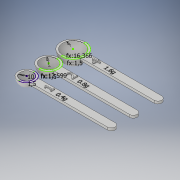
# Autodesk Inventor part: Pigmentlöffel
Saved by Autodesk Inventor 2018.2 (Build 222227000, 227)
## iProperties
Created: 2018-01-23
Part Number: Pigmentlöffel
Material: Generisch
Document SubType Name: Modeling
Designer: JochenAlt
Density: 1 g/cm^3
Appearance: Vorgabe
Author: JochenAlt
Autodesk Inventor part; units mm, degrees
ref_plane "XZ Plane" through (0, 0, 0) normal (0, 1, 0) x (-1, 0, 0)
ref_plane "XY Plane" through (0, 0, 0) normal (0, 0, 1) x (1, 0, 0)
sketch "Skizze1" plane through (0, 0, 0) normal (0, 0, 1) x (1, 0, 0)
  arc A0 (0, -5) -> (0, 5) centre (0, 0) ccw
  arc A1 (0, -6.5) -> (0, 6.5) centre (0, 0) ccw
  line L0 (0, -6.5) -> (0, -5)
  line L1 (0, 5) -> (0, 6.5)
  arc A2 (0, 11.07) -> (0, 23.669) centre (0, 17.3695) ccw
  arc A3 (0, 9.57) -> (0, 25.169) centre (0, 17.3695) ccw
  arc A4 (0, 28.5978) -> (0, 44.9639) centre (0, 36.7809) ccw
  arc A5 (0, 27.0978) -> (0, 46.4639) centre (0, 36.7809) ccw
  line L2 (0, 44.9639) -> (0, 46.4639)
  line L3 (0, 27.0978) -> (0, 28.5978)
  line L4 (0, 9.57) -> (0, 11.07)
  line L5 (0, 23.669) -> (0, 25.169)
  dimension "d0" = 10
  dimension "d8" = 1.5
  dimension "d9" = 12.599
  dimension "d10" = 1.5
  dimension "d11" = 16.3661
  dimension "d12" = 1.5
  constraints: 12 end point, 12 point on circle, 6 centre point, 6 vertical, 4 coincident
  measures "d0" diameter of A0
  measures "d8" radial gap between concentric circles of A1 A0
  measures "d9" diameter of A2
  measures "d10" radial gap between concentric circles of A3 A2
  measures "d11" diameter of A4
  measures "d12" radial gap between concentric circles of A5 A4
revolve "Umdrehung1" add sketch "Skizze1" angle 180 about axis through (0, -6.5, 0) along (0, 1, 0) contours A0 L1 A1 L0
revolve "Umdrehung2" add sketch "Skizze1" angle 180 about axis through (0, 9.57, 0) along (0, 1, 0) contours A2 L5 A3 L4
revolve "Umdrehung3" add sketch "Skizze1" angle 180 about axis through (0, 27.0978, 0) along (0, 1, 0) contours A4 L2 A5 L3
ref_plane "Arbeitsebene1" through (70, 0, 0) normal (1, 0, 0) x (0, 1, 0)
sketch "Skizze3" plane through (70, 0, 0) normal (1, 0, 0) x (0, 1, 0)
  line L0 (-5, 0) -> (5, 0) projected
  line L1 (-3, 0) -> (3, 0)
  line L2 (3, 0) -> (3, -2)
  line L3 (3, -2) -> (-3, -2)
  line L4 (-3, -2) -> (-3, 0)
  line L5 (14.3695, 0) -> (20.3695, 0)
  line L6 (20.3695, 0) -> (20.3695, -2)
  line L7 (20.3695, -2) -> (14.3695, -2)
  line L8 (14.3695, -2) -> (14.3695, 0)
  line L9 (33.7809, 0) -> (39.7809, 0)
  line L10 (39.7809, 0) -> (39.7809, -2)
  line L11 (39.7809, -2) -> (33.7809, -2)
  line L12 (33.7809, -2) -> (33.7809, 0)
  line L13 (25.169, 0) -> (9.57, 0) construction
  line L14 (46.4639, 0) -> (27.0978, 0) construction
  arc A0 (-5, 0) -> (5, 0) centre (0, 0) ccw construction
  line L15 (6.5, 0) -> (-6.5, 0) construction
  line L16 (0, 1.9354) -> (0, -11.6125) construction
  line L17 (-17.0928, 0) -> (57.0567, 0) construction
  line L18 (36.7809, 0) -> (36.7809, -9.6771) construction
  line L19 (17.3695, 0) -> (17.3695, -7.848) construction
  dimension "d16" = 2
  dimension "d17" = 6
  dimension "d21" = 6
  dimension "d22" = 6
  constraints: 28 end point, 6 parallel, 3 coincident, 3 horizontal, 3 perpendicular, 3 point on line, 2 collinear, 2 vertical, 4 other
  measures "d16" distance of the line from the sketch origin of L3
  measures "d17" distance between parallel lines of L2 L4
  measures "d21" distance between parallel lines of L6 L8
  measures "d22" distance between parallel lines of L10 L12
extrude "Extrusion2" add sketch "Skizze3" against normal up to next
fillet "Rundung1" radius 3 6 edges at (70, 3, -1) (70, -3, -1) (70, 14.3695, -1) (70, 20.3695, -1) (70, 33.7809, -1) (70, 39.7809, -1)
sketch "Skizze5" plane through (0, 0, 0) normal (0, 0, 1) x (1, 0, 0)
  line L0 (20.5874, 1.818) -> (20.5874, -1.1578)
  line L1 (20.5874, -1.1578) -> (19.9646, -1.1578)
  line L2 (19.9646, -1.1578) -> (19.9646, -0.0505)
  line L3 (19.9646, -0.0505) -> (15.8765, -0.0505)
  line L4 (15.8765, -0.0505) -> (15.8765, -1.1578)
  line L5 (15.8765, -1.1578) -> (15.3179, -1.1578)
  spline S0 degree 2 poles (15.3179, -1.1578) (15.3179, -0.53) (14.962, 0.0632) (14.4677, 0.1027) knots 0 0 0 1 2 2 2
  line L6 (14.4677, 0.1027) -> (14.4677, 0.7354)
  line L7 (14.4677, 0.7354) -> (19.9646, 0.7354)
  line L8 (19.9646, 0.7354) -> (19.9646, 1.818)
  line L9 (19.9646, 1.818) -> (20.5874, 1.818)
  line L10 (20.8624, 19.5576) -> (20.8624, 15.7958)
  line L11 (20.8624, 15.7958) -> (19.9973, 15.7958)
  spline S1 degree 2 poles (19.9973, 15.7958) (19.6167, 16.2012) (18.9098, 16.9229) (18.5292, 17.2689) knots 0 0 0 1 2 2 2
  spline S2 degree 2 poles (18.5292, 17.2689) (17.763, 17.9659) (16.8435, 18.4751) (16.3541, 18.4751) knots 0 0 0 1 2 2 2
  spline S3 degree 2 poles (16.3541, 18.4751) (16.0971, 18.4751) (15.7115, 18.3169) (15.5879, 18.1735) knots 0 0 0 1 2 2 2
  spline S4 degree 2 poles (15.5879, 18.1735) (15.4643, 18.0302) (15.3408, 17.6545) (15.3408, 17.4271) knots 0 0 0 1 2 2 2
  spline S5 degree 2 poles (15.3408, 17.4271) (15.3408, 17.2096) (15.4495, 16.7647) (15.5335, 16.562) knots 0 0 0 1 2 2 2
  spline S6 degree 2 poles (15.5335, 16.562) (15.6027, 16.389) (15.8005, 16.0677) (15.8697, 15.9688) knots 0 0 0 1 2 2 2
  line L12 (15.8697, 15.9688) -> (15.8697, 15.9243)
  line L13 (15.8697, 15.9243) -> (14.9997, 15.9243)
  spline S7 degree 2 poles (14.9997, 15.9243) (14.8761, 16.1764) (14.6339, 17.0811) (14.6339, 17.4864) knots 0 0 0 1 2 2 2
  spline S8 degree 2 poles (14.6339, 17.4864) (14.6339, 18.3416) (15.5385, 19.3055) (16.3096, 19.3055) knots 0 0 0 1 2 2 2
  spline S9 degree 2 poles (16.3096, 19.3055) (16.6705, 19.3055) (17.2736, 19.1375) (17.5306, 18.9892) knots 0 0 0 1 2 2 2
  spline S10 degree 2 poles (17.5306, 18.9892) (17.7976, 18.8409) (18.3215, 18.4108) (18.5737, 18.1735) knots 0 0 0 1 2 2 2
  spline S11 degree 2 poles (18.5737, 18.1735) (18.9938, 17.7879) (19.8935, 16.8438) (20.1555, 16.562) knots 0 0 0 1 2 2 2
  line L14 (20.1555, 16.562) -> (20.1555, 19.5576)
  line L15 (20.1555, 19.5576) -> (20.8624, 19.5576)
  line L16 (18.4703, 38.8851) -> (18.4703, 38.1585)
  line L17 (18.4703, 38.1585) -> (20.5663, 38.1585)
  line L18 (20.5663, 38.1585) -> (20.5663, 37.3725)
  line L19 (20.5663, 37.3725) -> (18.4703, 37.3725)
  line L20 (18.4703, 37.3725) -> (18.4703, 34.6784)
  line L21 (18.4703, 34.6784) -> (17.6102, 34.6784)
  line L22 (17.6102, 34.6784) -> (14.4663, 37.4071)
  line L23 (14.4663, 37.4071) -> (14.4663, 38.1585)
  line L24 (14.4663, 38.1585) -> (17.8129, 38.1585)
  line L25 (17.8129, 38.1585) -> (17.8129, 38.8851)
  line L26 (17.8129, 38.8851) -> (18.4703, 38.8851)
  line L27 (17.8129, 37.3725) -> (15.4302, 37.3725)
  line L28 (15.4302, 37.3725) -> (17.8129, 35.321)
  line L29 (17.8129, 35.321) -> (17.8129, 37.3725)
  spline S12 degree 2 poles (26.2288, -0.1714) (26.2288, -0.9915) (25.7521, -1.7597) (25.2556, -1.7597) knots 0 0 0 1 2 2 2
  spline S13 degree 2 poles (25.2556, -1.7597) (24.7517, -1.7597) (24.28, -0.9767) (24.28, -0.1739) knots 0 0 0 1 2 2 2
  spline S14 degree 2 poles (24.28, -0.1739) (24.28, 0.6511) (24.7567, 1.4143) (25.2556, 1.4143) knots 0 0 0 1 2 2 2
  spline S15 degree 2 poles (25.2556, 1.4143) (25.757, 1.4143) (26.2288, 0.6239) (26.2288, -0.1714) knots 0 0 0 1 2 2 2
  spline S16 degree 2 poles (25.7052, -1.1002) (25.7644, -0.9495) (25.8138, -0.4851) (25.8138, -0.1714) knots 0 0 0 1 2 2 2
  spline S17 degree 2 poles (25.8138, -0.1714) (25.8138, 0.1423) (25.7644, 0.6042) (25.7027, 0.7598) knots 0 0 0 1 2 2 2
  spline S18 degree 2 poles (25.7027, 0.7598) (25.6409, 0.9154) (25.426, 1.0759) (25.2556, 1.0759) knots 0 0 0 1 2 2 2
  spline S19 degree 2 poles (25.2556, 1.0759) (25.0852, 1.0759) (24.8654, 0.9154) (24.8011, 0.7548) knots 0 0 0 1 2 2 2
  spline S20 degree 2 poles (24.8011, 0.7548) (24.7394, 0.5992) (24.6949, 0.125) (24.6949, -0.1739) knots 0 0 0 1 2 2 2
  spline S21 degree 2 poles (24.6949, -0.1739) (24.6949, -0.495) (24.7344, -0.9248) (24.7987, -1.0927) knots 0 0 0 1 2 2 2
  spline S22 degree 2 poles (24.7987, -1.0927) (24.8579, -1.2508) (25.0778, -1.4213) (25.2556, -1.4213) knots 0 0 0 1 2 2 2
  spline S23 degree 2 poles (25.2556, -1.4213) (25.4236, -1.4213) (25.6434, -1.2607) (25.7052, -1.1002) knots 0 0 0 1 2 2 2
  line L30 (27.2736, -1.6954) -> (26.7846, -1.6954)
  line L31 (26.7846, -1.6954) -> (26.7846, -1.1125)
  line L32 (26.7846, -1.1125) -> (27.2736, -1.1125)
  line L33 (27.2736, -1.1125) -> (27.2736, -1.6954)
  line L34 (29.8498, -0.6481) -> (29.4868, -0.6481)
  line L35 (29.4868, -0.6481) -> (29.4868, -1.6954)
  line L36 (29.4868, -1.6954) -> (29.094, -1.6954)
  line L37 (29.094, -1.6954) -> (29.094, -0.6481)
  line L38 (29.094, -0.6481) -> (27.7479, -0.6481)
  line L39 (27.7479, -0.6481) -> (27.7479, -0.2184)
  line L40 (27.7479, -0.2184) -> (29.1113, 1.3526)
  line L41 (29.1113, 1.3526) -> (29.4868, 1.3526)
  line L42 (29.4868, 1.3526) -> (29.4868, -0.3196)
  line L43 (29.4868, -0.3196) -> (29.8498, -0.3196)
  line L44 (29.8498, -0.3196) -> (29.8498, -0.6481)
  line L45 (29.094, -0.3196) -> (29.094, 0.8709)
  line L46 (29.094, 0.8709) -> (28.069, -0.3196)
  line L47 (28.069, -0.3196) -> (29.094, -0.3196)
  spline S24 degree 2 poles (30.3142, -2.061) (30.3537, -2.0783) (30.5044, -2.1326) (30.6007, -2.1549) knots 0 0 0 1 2 2 2
  spline S25 degree 2 poles (30.6007, -2.1549) (30.7069, -2.182) (30.8873, -2.2141) (30.9935, -2.2141) knots 0 0 0 1 2 2 2
  spline S26 degree 2 poles (30.9935, -2.2141) (31.1713, -2.2141) (31.4183, -2.1203) (31.4875, -2.0363) knots 0 0 0 1 2 2 2
  spline S27 degree 2 poles (31.4875, -2.0363) (31.5542, -1.9523) (31.606, -1.7325) (31.606, -1.5917) knots 0 0 0 1 2 2 2
  line L48 (31.606, -1.5917) -> (31.606, -1.3916)
  spline S28 degree 2 poles (31.606, -1.3916) (31.4504, -1.5275) (31.1515, -1.6559) (30.9268, -1.6559) knots 0 0 0 1 2 2 2
  spline S29 degree 2 poles (30.9268, -1.6559) (30.5365, -1.6559) (30.0746, -1.0755) (30.0746, -0.5296) knots 0 0 0 1 2 2 2
  spline S30 degree 2 poles (30.0746, -0.5296) (30.0746, -0.2455) (30.2352, 0.1941) (30.3685, 0.3497) knots 0 0 0 1 2 2 2
  spline S31 degree 2 poles (30.3685, 0.3497) (30.497, 0.4955) (30.8502, 0.656) (31.0379, 0.656) knots 0 0 0 1 2 2 2
  spline S32 degree 2 poles (31.0379, 0.656) (31.2158, 0.656) (31.4751, 0.572) (31.606, 0.4955) knots 0 0 0 1 2 2 2
  line L49 (31.606, 0.4955) -> (31.6283, 0.5918)
  line L50 (31.6283, 0.5918) -> (31.9914, 0.5918)
  line L51 (31.9914, 0.5918) -> (31.9914, -1.4336)
  spline S33 degree 2 poles (31.9914, -1.4336) (31.9914, -2.0165) (31.485, -2.5599) (30.9638, -2.5599) knots 0 0 0 1 2 2 2
  spline S34 degree 2 poles (30.9638, -2.5599) (30.7959, -2.5599) (30.4451, -2.5056) (30.2944, -2.4611) knots 0 0 0 1 2 2 2
  line L52 (30.2944, -2.4611) -> (30.2944, -2.061)
  line L53 (30.2944, -2.061) -> (30.3142, -2.061)
  line L54 (31.606, -1.0755) -> (31.606, 0.1818)
  spline S35 degree 2 poles (31.606, 0.1818) (31.4628, 0.2509) (31.2207, 0.3102) (31.0997, 0.3102) knots 0 0 0 1 2 2 2
  spline S36 degree 2 poles (31.0997, 0.3102) (30.8082, 0.3102) (30.4723, -0.1196) (30.4723, -0.5222) knots 0 0 0 1 2 2 2
  spline S37 degree 2 poles (30.4723, -0.5222) (30.4723, -0.9026) (30.7267, -1.3002) (31.0132, -1.3002) knots 0 0 0 1 2 2 2
  spline S38 degree 2 poles (31.0132, -1.3002) (31.1639, -1.3002) (31.4801, -1.1817) (31.606, -1.0755) knots 0 0 0 1 2 2 2
  spline S39 degree 2 poles (25.8845, 17.2087) (25.8845, 16.3887) (25.4078, 15.6205) (24.9113, 15.6205) knots 0 0 0 1 2 2 2
  spline S40 degree 2 poles (24.9113, 15.6205) (24.4074, 15.6205) (23.9357, 16.4035) (23.9357, 17.2062) knots 0 0 0 1 2 2 2
  spline S41 degree 2 poles (23.9357, 17.2062) (23.9357, 18.0312) (24.4124, 18.7945) (24.9113, 18.7945) knots 0 0 0 1 2 2 2
  spline S42 degree 2 poles (24.9113, 18.7945) (25.4127, 18.7945) (25.8845, 18.004) (25.8845, 17.2087) knots 0 0 0 1 2 2 2
  spline S43 degree 2 poles (25.3609, 16.28) (25.4201, 16.4306) (25.4695, 16.895) (25.4695, 17.2087) knots 0 0 0 1 2 2 2
  spline S44 degree 2 poles (25.4695, 17.2087) (25.4695, 17.5224) (25.4201, 17.9843) (25.3584, 18.1399) knots 0 0 0 1 2 2 2
  spline S45 degree 2 poles (25.3584, 18.1399) (25.2966, 18.2955) (25.0818, 18.4561) (24.9113, 18.4561) knots 0 0 0 1 2 2 2
  spline S46 degree 2 poles (24.9113, 18.4561) (24.7409, 18.4561) (24.5211, 18.2955) (24.4568, 18.135) knots 0 0 0 1 2 2 2
  spline S47 degree 2 poles (24.4568, 18.135) (24.3951, 17.9793) (24.3506, 17.5051) (24.3506, 17.2062) knots 0 0 0 1 2 2 2
  spline S48 degree 2 poles (24.3506, 17.2062) (24.3506, 16.8851) (24.3902, 16.4553) (24.4544, 16.2874) knots 0 0 0 1 2 2 2
  spline S49 degree 2 poles (24.4544, 16.2874) (24.5137, 16.1293) (24.7335, 15.9589) (24.9113, 15.9589) knots 0 0 0 1 2 2 2
  spline S50 degree 2 poles (24.9113, 15.9589) (25.0793, 15.9589) (25.2991, 16.1194) (25.3609, 16.28) knots 0 0 0 1 2 2 2
  line L55 (26.9293, 15.6847) -> (26.4403, 15.6847)
  line L56 (26.4403, 15.6847) -> (26.4403, 16.2676)
  line L57 (26.4403, 16.2676) -> (26.9293, 16.2676)
  line L58 (26.9293, 16.2676) -> (26.9293, 15.6847)
  spline S51 degree 2 poles (28.4657, 15.6155) (28.2384, 15.6155) (27.8655, 15.7514) (27.7346, 15.8774) knots 0 0 0 1 2 2 2
  spline S52 degree 2 poles (27.7346, 15.8774) (27.6061, 16.0009) (27.4727, 16.3368) (27.4727, 16.527) knots 0 0 0 1 2 2 2
  spline S53 degree 2 poles (27.4727, 16.527) (27.4727, 16.774) (27.737, 17.1889) (27.989, 17.3124) knots 0 0 0 1 2 2 2
  line L59 (27.989, 17.3124) -> (27.989, 17.3248)
  spline S54 degree 2 poles (27.989, 17.3248) (27.7642, 17.4557) (27.5468, 17.7669) (27.5468, 17.9991) knots 0 0 0 1 2 2 2
  spline S55 degree 2 poles (27.5468, 17.9991) (27.5468, 18.3424) (28.0655, 18.8019) (28.4657, 18.8019) knots 0 0 0 1 2 2 2
  spline S56 degree 2 poles (28.4657, 18.8019) (28.8806, 18.8019) (29.3821, 18.3671) (29.3821, 18.0263) knots 0 0 0 1 2 2 2
  spline S57 degree 2 poles (29.3821, 18.0263) (29.3821, 17.8213) (29.1425, 17.4211) (28.9177, 17.3075) knots 0 0 0 1 2 2 2
  line L60 (28.9177, 17.3075) -> (28.9177, 17.2952)
  spline S58 degree 2 poles (28.9177, 17.2952) (29.1845, 17.1717) (29.4586, 16.816) (29.4586, 16.5344) knots 0 0 0 1 2 2 2
  spline S59 degree 2 poles (29.4586, 16.5344) (29.4586, 16.1441) (28.8905, 15.6155) (28.4657, 15.6155) knots 0 0 0 1 2 2 2
  spline S60 degree 2 poles (29.0387, 16.4949) (29.0387, 16.6826) (28.8905, 16.9049) (28.6806, 17.0185) knots 0 0 0 1 2 2 2
  spline S61 degree 2 poles (28.6806, 17.0185) (28.6114, 17.058) (28.3792, 17.1494) (28.2335, 17.2087) knots 0 0 0 1 2 2 2
  spline S62 degree 2 poles (28.2335, 17.2087) (28.0655, 17.0976) (27.8852, 16.7666) (27.8852, 16.5566) knots 0 0 0 1 2 2 2
  spline S63 degree 2 poles (27.8852, 16.5566) (27.8852, 16.28) (28.2187, 15.9194) (28.4706, 15.9194) knots 0 0 0 1 2 2 2
  spline S64 degree 2 poles (28.4706, 15.9194) (28.7275, 15.9194) (29.0387, 16.2281) (29.0387, 16.4949) knots 0 0 0 1 2 2 2
  spline S65 degree 2 poles (28.9819, 18.0213) (28.9819, 18.2263) (28.7077, 18.5005) (28.4632, 18.5005) knots 0 0 0 1 2 2 2
  spline S66 degree 2 poles (28.4632, 18.5005) (28.2409, 18.5005) (27.9569, 18.256) (27.9569, 18.046) knots 0 0 0 1 2 2 2
  spline S67 degree 2 poles (27.9569, 18.046) (27.9569, 17.8954) (28.1026, 17.6854) (28.2483, 17.6014) knots 0 0 0 1 2 2 2
  spline S68 degree 2 poles (28.2483, 17.6014) (28.3101, 17.5669) (28.5719, 17.4458) (28.6781, 17.4112) knots 0 0 0 1 2 2 2
  spline S69 degree 2 poles (28.6781, 17.4112) (28.8559, 17.5471) (28.9819, 17.8361) (28.9819, 18.0213) knots 0 0 0 1 2 2 2
  spline S70 degree 2 poles (29.9699, 15.3191) (30.0094, 15.3018) (30.1601, 15.2475) (30.2564, 15.2253) knots 0 0 0 1 2 2 2
  spline S71 degree 2 poles (30.2564, 15.2253) (30.3627, 15.1981) (30.543, 15.166) (30.6492, 15.166) knots 0 0 0 1 2 2 2
  spline S72 degree 2 poles (30.6492, 15.166) (30.827, 15.166) (31.074, 15.2599) (31.1432, 15.3438) knots 0 0 0 1 2 2 2
  spline S73 degree 2 poles (31.1432, 15.3438) (31.2099, 15.4278) (31.2617, 15.6477) (31.2617, 15.7884) knots 0 0 0 1 2 2 2
  line L61 (31.2617, 15.7884) -> (31.2617, 15.9885)
  spline S74 degree 2 poles (31.2617, 15.9885) (31.1061, 15.8527) (30.8073, 15.7242) (30.5825, 15.7242) knots 0 0 0 1 2 2 2
  spline S75 degree 2 poles (30.5825, 15.7242) (30.1922, 15.7242) (29.7303, 16.3047) (29.7303, 16.8505) knots 0 0 0 1 2 2 2
  spline S76 degree 2 poles (29.7303, 16.8505) (29.7303, 17.1346) (29.8909, 17.5743) (30.0243, 17.7299) knots 0 0 0 1 2 2 2
  spline S77 degree 2 poles (30.0243, 17.7299) (30.1527, 17.8756) (30.5059, 18.0362) (30.6936, 18.0362) knots 0 0 0 1 2 2 2
  spline S78 degree 2 poles (30.6936, 18.0362) (30.8715, 18.0362) (31.1308, 17.9522) (31.2617, 17.8756) knots 0 0 0 1 2 2 2
  line L62 (31.2617, 17.8756) -> (31.284, 17.9719)
  line L63 (31.284, 17.9719) -> (31.6471, 17.9719)
  line L64 (31.6471, 17.9719) -> (31.6471, 15.9465)
  spline S79 degree 2 poles (31.6471, 15.9465) (31.6471, 15.3636) (31.1407, 14.8202) (30.6195, 14.8202) knots 0 0 0 1 2 2 2
  spline S80 degree 2 poles (30.6195, 14.8202) (30.4516, 14.8202) (30.1008, 14.8745) (29.9502, 14.919) knots 0 0 0 1 2 2 2
  line L65 (29.9502, 14.919) -> (29.9502, 15.3191)
  line L66 (29.9502, 15.3191) -> (29.9699, 15.3191)
  line L67 (31.2617, 16.3047) -> (31.2617, 17.5619)
  spline S81 degree 2 poles (31.2617, 17.5619) (31.1185, 17.6311) (30.8764, 17.6904) (30.7554, 17.6904) knots 0 0 0 1 2 2 2
  spline S82 degree 2 poles (30.7554, 17.6904) (30.4639, 17.6904) (30.128, 17.2606) (30.128, 16.858) knots 0 0 0 1 2 2 2
  spline S83 degree 2 poles (30.128, 16.858) (30.128, 16.4776) (30.3824, 16.0799) (30.6689, 16.0799) knots 0 0 0 1 2 2 2
  spline S84 degree 2 poles (30.6689, 16.0799) (30.8196, 16.0799) (31.1358, 16.1985) (31.2617, 16.3047) knots 0 0 0 1 2 2 2
  line L68 (26.9061, 35.4531) -> (25.4192, 35.4531)
  line L69 (25.4192, 35.4531) -> (25.4192, 35.7643)
  line L70 (25.4192, 35.7643) -> (25.9725, 35.7643)
  line L71 (25.9725, 35.7643) -> (25.9725, 37.807)
  line L72 (25.9725, 37.807) -> (25.4192, 37.807)
  line L73 (25.4192, 37.807) -> (25.4192, 38.0861)
  spline S85 degree 2 poles (25.4192, 38.0861) (25.7329, 38.0861) (26.0293, 38.264) (26.049, 38.511) knots 0 0 0 1 2 2 2
  line L74 (26.049, 38.511) -> (26.3652, 38.511)
  line L75 (26.3652, 38.511) -> (26.3652, 35.7643)
  line L76 (26.3652, 35.7643) -> (26.9061, 35.7643)
  line L77 (26.9061, 35.7643) -> (26.9061, 35.4531)
  line L78 (28.1214, 35.4531) -> (27.6323, 35.4531)
  line L79 (27.6323, 35.4531) -> (27.6323, 36.036)
  line L80 (27.6323, 36.036) -> (28.1214, 36.036)
  line L81 (28.1214, 36.036) -> (28.1214, 35.4531)
  spline S86 degree 2 poles (30.663, 36.4411) (30.663, 36.2065) (30.5074, 35.8088) (30.3765, 35.6754) knots 0 0 0 1 2 2 2
  spline S87 degree 2 poles (30.3765, 35.6754) (30.2406, 35.5346) (29.8998, 35.3889) (29.6948, 35.3889) knots 0 0 0 1 2 2 2
  spline S88 degree 2 poles (29.6948, 35.3889) (29.4898, 35.3889) (29.1514, 35.5272) (29.0229, 35.6655) knots 0 0 0 1 2 2 2
  spline S89 degree 2 poles (29.0229, 35.6655) (28.8648, 35.831) (28.687, 36.3868) (28.687, 36.7919) knots 0 0 0 1 2 2 2
  spline S90 degree 2 poles (28.687, 36.7919) (28.687, 37.1895) (28.85, 37.8293) (29.0205, 38.0664) knots 0 0 0 1 2 2 2
  spline S91 degree 2 poles (29.0205, 38.0664) (29.1859, 38.2986) (29.7096, 38.5579) (30.0529, 38.5579) knots 0 0 0 1 2 2 2
  spline S92 degree 2 poles (30.0529, 38.5579) (30.1542, 38.5579) (30.332, 38.5382) (30.3987, 38.5159) knots 0 0 0 1 2 2 2
  line L82 (30.3987, 38.5159) -> (30.3987, 38.1232)
  line L83 (30.3987, 38.1232) -> (30.3814, 38.1232)
  spline S93 degree 2 poles (30.3814, 38.1232) (30.3246, 38.1528) (30.1171, 38.2047) (29.9986, 38.2047) knots 0 0 0 1 2 2 2
  spline S94 degree 2 poles (29.9986, 38.2047) (29.6182, 38.2047) (29.1514, 37.6909) (29.1069, 37.1871) knots 0 0 0 1 2 2 2
  spline S95 degree 2 poles (29.1069, 37.1871) (29.2526, 37.2883) (29.5589, 37.3995) (29.7417, 37.3995) knots 0 0 0 1 2 2 2
  spline S96 degree 2 poles (29.7417, 37.3995) (29.9195, 37.3995) (30.1863, 37.3279) (30.332, 37.2192) knots 0 0 0 1 2 2 2
  spline S97 degree 2 poles (30.332, 37.2192) (30.5, 37.0932) (30.663, 36.7029) (30.663, 36.4411) knots 0 0 0 1 2 2 2
  spline S98 degree 2 poles (30.2481, 36.4238) (30.2481, 36.6115) (30.1493, 36.866) (30.0406, 36.9549) knots 0 0 0 1 2 2 2
  spline S99 degree 2 poles (30.0406, 36.9549) (29.9591, 37.0191) (29.7565, 37.0611) (29.6503, 37.0611) knots 0 0 0 1 2 2 2
  spline S100 degree 2 poles (29.6503, 37.0611) (29.507, 37.0611) (29.2378, 36.9746) (29.1069, 36.8931) knots 0 0 0 1 2 2 2
  spline S101 degree 2 poles (29.1069, 36.8931) (29.1044, 36.8487) (29.0995, 36.7647) (29.0995, 36.7005) knots 0 0 0 1 2 2 2
  spline S102 degree 2 poles (29.0995, 36.7005) (29.0995, 36.3843) (29.223, 35.9965) (29.3169, 35.8952) knots 0 0 0 1 2 2 2
  spline S103 degree 2 poles (29.3169, 35.8952) (29.4033, 35.7989) (29.591, 35.7223) (29.6972, 35.7223) knots 0 0 0 1 2 2 2
  spline S104 degree 2 poles (29.6972, 35.7223) (29.9442, 35.7223) (30.2481, 36.0731) (30.2481, 36.4238) knots 0 0 0 1 2 2 2
  spline S105 degree 2 poles (31.162, 35.0875) (31.2015, 35.0703) (31.3522, 35.0159) (31.4485, 34.9937) knots 0 0 0 1 2 2 2
  spline S106 degree 2 poles (31.4485, 34.9937) (31.5547, 34.9665) (31.735, 34.9344) (31.8412, 34.9344) knots 0 0 0 1 2 2 2
  spline S107 degree 2 poles (31.8412, 34.9344) (32.0191, 34.9344) (32.2661, 35.0283) (32.3352, 35.1122) knots 0 0 0 1 2 2 2
  spline S108 degree 2 poles (32.3352, 35.1122) (32.4019, 35.1962) (32.4538, 35.4161) (32.4538, 35.5568) knots 0 0 0 1 2 2 2
  line L84 (32.4538, 35.5568) -> (32.4538, 35.7569)
  spline S109 degree 2 poles (32.4538, 35.7569) (32.2982, 35.6211) (31.9993, 35.4926) (31.7745, 35.4926) knots 0 0 0 1 2 2 2
  spline S110 degree 2 poles (31.7745, 35.4926) (31.3843, 35.4926) (30.9224, 36.0731) (30.9224, 36.619) knots 0 0 0 1 2 2 2
  spline S111 degree 2 poles (30.9224, 36.619) (30.9224, 36.903) (31.0829, 37.3427) (31.2163, 37.4983) knots 0 0 0 1 2 2 2
  spline S112 degree 2 poles (31.2163, 37.4983) (31.3447, 37.644) (31.698, 37.8046) (31.8857, 37.8046) knots 0 0 0 1 2 2 2
  spline S113 degree 2 poles (31.8857, 37.8046) (32.0635, 37.8046) (32.3229, 37.7206) (32.4538, 37.644) knots 0 0 0 1 2 2 2
  line L85 (32.4538, 37.644) -> (32.476, 37.7403)
  line L86 (32.476, 37.7403) -> (32.8391, 37.7403)
  line L87 (32.8391, 37.7403) -> (32.8391, 35.7149)
  spline S114 degree 2 poles (32.8391, 35.7149) (32.8391, 35.132) (32.3327, 34.5886) (31.8116, 34.5886) knots 0 0 0 1 2 2 2
  spline S115 degree 2 poles (31.8116, 34.5886) (31.6436, 34.5886) (31.2929, 34.6429) (31.1422, 34.6874) knots 0 0 0 1 2 2 2
  line L88 (31.1422, 34.6874) -> (31.1422, 35.0875)
  line L89 (31.1422, 35.0875) -> (31.162, 35.0875)
  line L90 (32.4538, 36.0731) -> (32.4538, 37.3303)
  spline S116 degree 2 poles (32.4538, 37.3303) (32.3105, 37.3995) (32.0685, 37.4588) (31.9474, 37.4588) knots 0 0 0 1 2 2 2
  spline S117 degree 2 poles (31.9474, 37.4588) (31.656, 37.4588) (31.32, 37.029) (31.32, 36.6264) knots 0 0 0 1 2 2 2
  spline S118 degree 2 poles (31.32, 36.6264) (31.32, 36.246) (31.5745, 35.8483) (31.861, 35.8483) knots 0 0 0 1 2 2 2
  spline S119 degree 2 poles (31.861, 35.8483) (32.0116, 35.8483) (32.3278, 35.9669) (32.4538, 36.0731) knots 0 0 0 1 2 2 2
  point P0 (0, 0)
  point P1 (14.4677, -2.0822)
  point P2 (17.5163, 34.5153)
  point P3 (17.7481, 15.3509)
  point P4 (24.1095, 1.4143)
  point P5 (23.7652, 18.8019)
  point P6 (24.9573, 38.5579)
  constraints: 6 other
extrude "Extrusion4" add sketch "Skizze5" along normal blind 0.6 contours L0 L1 L2 L3 L4 L5 S0 L6 L7 L8 L9 | L10 L11 S1 S2 S3 S4 S5 S6 L12 L13 S7 S8 S9 S10 S11 L14 L15 | L16 L17 L18 L19 L20 L21 L22 L23 L24 L25 L26
extrude "Extrusion5" cut sketch "Skizze5" against normal blind 0.5 contours S12 S13 S14 S15 | L30 L31 L32 L33 | L34 L35 L36 L37 L38 L39 L40 L41 L42 L43 L44 | S24 S25 S26 S27 L48 S28 S29 S30 S31 S32 L49 L50 L51 S33 S34 L52 L53 | S39 S40 S41 S42 | L55 L56 L57 L58 | S51 S52 S53 L59 S54 S55 S56 S57 L60 S58 S59 | S70 S71 S72 S73 L61 S74 S75 S76 S77 S78 L62 L63 L64 S79 S80 L65 L66 | L68 L69 L70 L71 L72 L73 S85 L74 L75 L76 L77 | L78 L79 L80 L81 | S86 S87 S88 S89 S90 S91 S92 L82 L83 S93 S94 S95 S96 S97 | S105 S106 S107 S108 L84 S109 S110 S111 S112 S113 L85 L86 L87 S114 S115 L88 L89
equation "\"d9\" = 1.2599 * d0"
equation "\"d10\" = d8"
equation "\"d11\" = 1.299 * d9"
equation "\"d12\" = d10"
equation "\"d21\" = d17"
equation "\"d22\" = d17"
